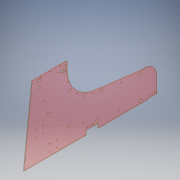
# Autodesk Inventor part: Storage Side Plate
Saved by Autodesk Inventor 2019.4 (Build 234330000, 330)
## iProperties
Created: 2020-01-11
Part Number: Storage Side Plate
Material: Polycarbonate, Smoke
Document SubType Name: Modeling
Designer: admin
Density: 1.2 g/cm^3
Appearance: Polycarbonate - Smoked
Mass: 1698.6 g
Surface Area: 5851.48 cm^2
Volume: 1415.5 cm^3
Author: admin
Autodesk Inventor part; units mm, degrees
ref_plane "YZ Plane" through (0, 0, 0) normal (1, 0, 0) x (0, 1, 0)
ref_plane "XZ Plane" through (0, 0, 0) normal (0, 1, 0) x (-1, 0, 0)
ref_plane "XY Plane" through (0, 0, 0) normal (0, 0, 1) x (1, 0, 0)
sketch "Sketch1" plane through (0, 0, 0) normal (1, 0, 0) x (0, 1, 0)
  arc A0 (273.7291, -166.7427) -> (45.384, -369.2015) centre (273.7291, -396.7427) ccw
  arc A1 (273.7291, 36.4573) -> (-156.3539, -344.8694) centre (273.7291, -396.7427) ccw
  line L0 (45.384, -369.2015) -> (9.2003, -669.2015)
  line L1 (-156.3539, -344.8694) -> (-192.5376, -644.8694)
  line L2 (48.9453, -381.4304) -> (48.9453, -441.4304)
  line L3 (-161.2547, -373.9304) -> (-161.2547, -293.9304)
  arc A2 (9.2003, -669.2015) -> (7.7612, -693.1504) centre (207.7612, -693.1504) ccw
  arc A3 (-192.5376, -644.8694) -> (-195.4388, -693.1504) centre (207.7612, -693.1504) ccw
  line L4 (-195.4388, -693.1504) -> (7.7612, -693.1504)
  line L5 (48.9453, -381.4304) -> (21.7149, -607.1979) construction
  line L6 (-161.2547, -373.9304) -> (-171.9549, -462.646) construction
  line L7 (273.7291, 36.4573) -> (323.7291, 36.4573)
  line L8 (323.7291, 36.4573) -> (323.7291, -166.7427)
  line L9 (323.7291, -166.7427) -> (273.7291, -166.7427)
  dimension "d4" = 203.2
  dimension "d6" = 5
  dimension "d7" = 1.3856
  dimension "d8" = 230
  dimension "d9" = 300
  dimension "d10" = 200
  dimension "d35" = 50
  constraints: 20 end point, 8 point on circle, 5 tangent, 4 centre point, 4 parallel, 2 coincident, 2 horizontal, 2 perpendicular, 1 line through centre
  measures "d4" distance of L7.start L9.end
  measures "d6" distance between parallel lines of L5 L0
  measures "d7" distance between parallel lines of L1 L6
  measures "d8" radius of A0
  measures "d9" vertical distance of L0.start L0.end
  measures "d10" radius of A2
  measures "d35" distance of L7.start L7.end
extrude "Extrusion1" add sketch "Sketch1" along normal blind 5
sketch "Sketch2" plane through (5, 0, 0) normal (1, 0, 0) x (0, 0, -1)
  line L0 (682.6743, -12.5697) -> (412.135, 20.0607) construction
  line L1 (412.135, 20.0607) -> (288.3305, 50.5351) construction
  line L2 (288.3305, 50.5351) -> (190.5511, 132.3607) construction
  line L3 (190.5511, 132.3607) -> (154.7427, 254.7291) construction
  circle A0 centre (682.6743, -12.5697) radius 9.5
  circle A1 centre (412.135, 20.0607) radius 9.5
  circle A2 centre (288.3305, 50.5351) radius 9.5
  circle A3 centre (190.5511, 132.3607) radius 9.5
  circle A4 centre (154.7427, 254.7291) radius 9.5
  line L4 (669.2015, 9.2003) -> (369.2015, 45.384) construction
  circle A5 centre (434.3269, 202.816) radius 88.9 construction
  line L5 (288.3305, 50.5351) -> (296.252, 66.8436) construction
  arc A6 (166.7427, 273.7291) -> (369.2015, 45.384) centre (396.7427, 273.7291) ccw construction
  line L6 (190.5511, 132.3607) -> (207.0464, 143.6702) construction
  line L7 (682.7467, -176.9612) -> (377.4593, -140.1397) construction
  line L8 (377.4593, -140.1397) -> (183.9514, -80.4659) construction
  line L9 (183.9514, -80.4659) -> (41.2141, 63.1735) construction
  line L10 (41.2141, 63.1735) -> (-24.4573, 254.7291) construction
  circle A7 centre (682.7467, -176.9612) radius 9.5
  circle A8 centre (377.4593, -140.1397) radius 9.5
  circle A9 centre (183.9514, -80.4659) radius 9.5
  circle A10 centre (41.2141, 63.1735) radius 9.5
  circle A11 centre (-24.4573, 254.7291) radius 9.5
  line L11 (-24.4573, 254.7291) -> (154.7427, 254.7291) construction
  line L12 (344.8694, -156.3539) -> (644.8694, -192.5376) projected
  line L13 (41.2141, 63.1735) -> (24.0055, 52.9821) construction
  arc A12 (-36.4573, 273.7291) -> (344.8694, -156.3539) centre (396.7427, 273.7291) ccw projected
  line L14 (166.7427, 323.7291) -> (-36.4573, 323.7291) projected
  line L15 (693.1504, -195.4388) -> (693.1504, 7.7612) projected
  line L16 (183.9514, -80.4659) -> (173.6518, -97.6099) construction
  circle A13 centre (155.7427, 296.7291) radius 25.4 construction
  circle A14 centre (-25.4573, 296.7291) radius 25.4 construction
  circle A15 centre (155.7427, 296.7291) radius 9.5
  circle A16 centre (-25.4573, 296.7291) radius 9.5
  circle A17 centre (547.4047, 3.7455) radius 2.75
  circle A18 centre (530.103, -158.5505) radius 2.75
  circle A19 centre (280.7054, -110.3028) radius 2.75
  circle A20 centre (350.2327, 35.2979) radius 2.75
  circle A21 centre (239.4408, 91.4479) radius 2.75
  circle A22 centre (112.5828, -8.6462) radius 2.75
  circle A23 centre (8.3784, 158.9513) radius 2.75
  circle A24 centre (172.6469, 193.5449) radius 2.75
  line L17 (288.3305, 50.5351) -> (183.9514, -80.4659) construction
  point P0 (0, 0)
  dimension "d11" = 272.5
  dimension "d12" = 19
  dimension "d13" = 19
  dimension "d14" = 19
  dimension "d15" = 19
  dimension "d16" = 19
  dimension "d18" = 12
  dimension "d19" = 20
  dimension "d20" = 177.8
  dimension "d22" = 20
  dimension "d23" = 19
  dimension "d24" = 19
  dimension "d25" = 19
  dimension "d26" = 19
  dimension "d28" = 19
  dimension "d29" = 20
  dimension "d34" = 20
  dimension "d36" = 69
  dimension "d37" = 10.4037
  dimension "d38" = 20
  dimension "d39" = 202.5
  dimension "d40" = 127.5
  dimension "d41" = 307.5
  dimension "d42" = 202.5
  dimension "d43" = 202.5
  dimension "d44" = 127.5
  dimension "d46" = 127.5
  dimension "d49" = 12
  dimension "d50" = 50.8
  dimension "d51" = 50.8
  dimension "d52" = 27
  dimension "d53" = 27
  dimension "d54" = 11
  dimension "d55" = 11
  dimension "d56" = 19
  dimension "d57" = 19
  dimension "d58" = 5.5
  dimension "d59" = 5.5
  dimension "d60" = 5.5
  dimension "d61" = 5.5
  dimension "d62" = 5.5
  dimension "d63" = 5.5
  dimension "d64" = 5.5
  dimension "d65" = 5.5
  dimension "d109" = 167.5
  constraints: 28 end point, 23 centre point, 11 coincident, 8 midpoint, 4 line through centre, 4 point on circle, 1 horizontal, 1 parallel
  measures "d11" distance of L0.start L0.end
  measures "d12" diameter of A0
  measures "d13" diameter of A1
  measures "d14" diameter of A2
  measures "d15" diameter of A3
  measures "d16" diameter of A4
  measures "d18" horizontal distance of A6.start L11.end
  measures "d19" distance from line of L4 A1.centre
  measures "d20" diameter of A5
  measures "d22" distance of L6.start L6.end
  measures "d23" diameter of A7
  measures "d24" diameter of A8
  measures "d25" diameter of A9
  measures "d26" diameter of A10
  measures "d28" diameter of A11
  measures "d29" distance between parallel lines of L12 L7
  measures "d34" distance of L13.start L13.end
  measures "d36" distance from line of L14 L11.end
  measures "d37" distance from line of L15 L7.start
  measures "d38" distance of L16.start L16.end
  measures "d39" distance of L7.end L8.end
  measures "d40" distance of L0.end L1.end
  measures "d41" distance of L7.start L7.end
  measures "d42" distance of L8.end L9.end
  measures "d43" distance of L10.end L9.end
  measures "d44" distance of L1.end L2.end
  measures "d46" distance of L2.end L3.end
  measures "d49" horizontal distance of L14.end L10.end
  measures "d50" diameter of A13
  measures "d51" diameter of A14
  measures "d52" distance from line of L14 A13.centre
  measures "d53" distance from line of L14 A14.centre
  measures "d54" horizontal distance of L14.end A14.centre
  measures "d55" horizontal distance of L14.start A13.centre
  measures "d56" diameter of A15
  measures "d57" diameter of A16
  measures "d58" diameter of A17
  measures "d59" diameter of A18
  measures "d60" diameter of A19
  measures "d61" diameter of A20
  measures "d62" diameter of A21
  measures "d63" diameter of A22
  measures "d64" diameter of A23
  measures "d65" diameter of A24
  measures "d109" distance of L5.start L16.start
extrude "Extrusion2" cut sketch "Sketch2" against normal through all
sketch "Sketch3" plane through (5, 0, 0) normal (1, 0, 0) x (0, 0, -1)
  line L0 (166.7427, 323.7291) -> (-36.4573, 323.7291) projected
  line L1 (-36.4573, 323.7291) -> (-76.4573, 323.7291)
  line L2 (-76.4573, 323.7291) -> (-76.4573, -195.4388)
  arc A0 (644.8694, -192.5376) -> (693.1504, -195.4388) centre (693.1504, 207.7612) ccw projected
  line L3 (-76.4573, -195.4388) -> (693.1504, -195.4388)
  arc A1 (-36.4573, 273.7291) -> (344.8694, -156.3539) centre (396.7427, 273.7291) ccw projected
  line L4 (344.8694, -156.3539) -> (644.8694, -192.5376) projected
  line L5 (-36.4573, 323.7291) -> (-36.4573, 273.7291) projected
  point P0 (0, 0)
  dimension "d66" = 40
  constraints: 6 end point, 2 perpendicular, 1 horizontal, 1 tangent
  measures "d66" distance of L0.end L1.end
extrude "Extrusion3" add sketch "Sketch3" against normal up to surface (5 mm away)
sketch "Sketch4" plane through (5, 0, 0) normal (1, 0, 0) x (0, 0, -1)
  line L0 (299.6427, -195.4388) -> (385.6427, -195.4388)
  line L1 (385.6427, -195.4388) -> (385.6427, -163.2388)
  line L2 (385.6427, -163.2388) -> (299.6427, -163.2388)
  line L3 (299.6427, -163.2388) -> (299.6427, -195.4388)
  line L4 (-76.4573, 323.7291) -> (-76.4573, -195.4388) projected
  line L5 (-76.4573, -195.4388) -> (693.1504, -195.4388) projected
  point P0 (0, 0)
  dimension "d69" = 376.1
  dimension "d70" = 32.2
  dimension "d71" = 86
  constraints: 8 end point, 2 parallel, 1 collinear, 1 horizontal, 1 perpendicular
  measures "d69" distance between parallel lines of L3 L4
  measures "d70" distance of L2.end L0.start
  measures "d71" distance of L1.end L2.end
extrude "Extrusion4" cut sketch "Sketch4" against normal through all
fillet "Fillet1" radius 3 2 edges at (2.5, -163.2388, -299.6427) (2.5, -163.2388, -385.6427)
thicken "Thicken1" operation add thickness 2.2 both sides no extend neighbours yes toward (0, 1, 0) faces at (3.3333, -195.4388, -48.9094)
thicken "Thicken2" operation add thickness 2.2 both sides no extend neighbours yes toward (0, 1, 0) faces at (1.6667, -195.4388, -488.1453)
sketch "Sketch5" plane through (5, 0, 0) normal (1, 0, 0) x (0, 0, -1)
  line L0 (693.1504, 7.7612) -> (793.1504, 7.7612)
  line L1 (793.1504, 7.7612) -> (793.1504, -188.2388)
  line L2 (793.1504, -188.2388) -> (732.1504, -188.2388)
  line L3 (732.1504, -188.2388) -> (732.1504, -193.2388)
  line L4 (385.6427, -193.2388) -> (693.1504, -193.2388) projected
  line L5 (732.1504, -193.2388) -> (693.1504, -193.2388)
  line L6 (693.1504, -193.2388) -> (693.1504, 7.7612)
  point P0 (0, 0)
  dimension "d79" = 5
  dimension "d80" = 100
  dimension "d81" = 39
  constraints: 12 end point, 4 perpendicular, 1 horizontal, 1 vertical
  measures "d79" distance of L2.end L3.end
  measures "d80" distance of L0.start L0.end
  measures "d81" distance of L3.end L4.end
extrude "Extrusion5" add sketch "Sketch5" against normal up to surface (5 mm away)
fillet "Fillet2" radius 3 1 edges at (2.5, -188.2388, -732.1504)
fillet "Fillet3" radius 80 1 edges at (2.5, 7.7612, -793.1504)
sketch "Sketch6" plane through (0, 0, 0) normal (-1, 0, 0) x (0, 0, 1)
  circle A0 centre (-352.6427, -150.2388) radius 2.75 projected
  circle A1 centre (-332.6427, -150.2388) radius 2.75 projected
  circle A2 centre (-312.6427, -150.2388) radius 2.75 projected
  point P0 (0, 0)
extrude "Extrusion6" cut sketch "Sketch6" against normal through all
sketch "Sketch7" plane through (5, 0, 0) normal (1, 0, 0) x (0, 0, -1)
  circle A0 centre (743.1504, -175.2388) radius 2.75 projected
  circle A1 centre (763.1504, -175.2388) radius 2.75 projected
  circle A2 centre (783.1504, -175.2388) radius 2.75 projected
  point P0 (0, 0)
extrude "Extrusion7" cut sketch "Sketch7" against normal through all
sketch "Sketch8" plane through (5, 0, 0) normal (1, 0, 0) x (0, 0, -1)
  line L0 (166.7427, 323.7291) -> (-76.4573, 323.7291) projected
  line L1 (-76.4573, 323.7291) -> (-134.8573, -193.2388)
  line L2 (299.6427, -193.2388) -> (-76.4573, -193.2388) projected
  line L3 (-134.8573, -193.2388) -> (-76.4573, -193.2388)
  line L4 (-76.4573, -193.2388) -> (-76.4573, 323.7291)
  line L5 (-76.4573, -193.2388) -> (299.6427, -193.2388) projected
  point P0 (0, 0)
  dimension "d90" = 58.4
  constraints: 6 end point, 1 collinear, 1 perpendicular
  measures "d90" distance of L2.end L1.end
extrude "Extrusion8" add sketch "Sketch8" against normal up to surface (5 mm away)
sketch "Sketch9" plane through (5, 0, 0) normal (1, 0, 0) x (0, 0, -1)
  circle A0 centre (-16.4573, 313.7291) radius 2.75 projected
  circle A1 centre (53.5427, 313.7291) radius 2.75 projected
  circle A2 centre (123.5427, 313.7291) radius 2.75 projected
  circle A3 centre (312.6427, -150.2388) radius 2.75 projected
  circle A4 centre (332.6427, -150.2388) radius 2.75 projected
  circle A5 centre (352.6427, -150.2388) radius 2.75 projected
  circle A6 centre (743.1504, -175.2388) radius 2.75 projected
  circle A7 centre (763.1504, -175.2388) radius 2.75 projected
  circle A8 centre (783.1504, -175.2388) radius 2.75 projected
  point P0 (0, 0)
extrude "Extrusion9" cut sketch "Sketch9" against normal through all contours A0 | A1 | A2
sketch "Sketch10" plane through (5, 0, 0) normal (1, 0, 0) x (0, 0, -1)
  circle A0 centre (73.275, -143.7666) radius 9.5 construction
  circle A1 centre (183.9514, -80.4659) radius 9.5 projected
  line L0 (73.275, -143.7666) -> (183.9514, -80.4659) construction
  line L1 (-134.8573, -193.2388) -> (299.6427, -193.2388) projected
  line L2 (48.275, -168.7666) -> (98.275, -168.7666) construction
  line L3 (98.275, -168.7666) -> (98.275, -118.7666) construction
  line L4 (98.275, -118.7666) -> (48.275, -118.7666) construction
  line L5 (48.275, -118.7666) -> (48.275, -168.7666) construction
  line L6 (48.275, -168.7666) -> (98.275, -118.7666) construction
  line L7 (98.275, -168.7666) -> (48.275, -118.7666) construction
  circle A2 centre (48.275, -118.7666) radius 2.2
  circle A3 centre (98.275, -118.7666) radius 2.2
  circle A4 centre (48.275, -168.7666) radius 2.2
  circle A5 centre (98.275, -168.7666) radius 2.2
  circle A6 centre (190.5511, 132.3607) radius 9.5 projected
  line L8 (73.275, -143.7666) -> (190.5511, 132.3607) construction
  circle A7 centre (-25.4573, -10.7709) radius 9.5 construction
  line L9 (-50.4573, -35.7709) -> (-0.4573, -35.7709) construction
  line L10 (-0.4573, -35.7709) -> (-0.4573, 14.2291) construction
  line L11 (-0.4573, 14.2291) -> (-50.4573, 14.2291) construction
  line L12 (-50.4573, 14.2291) -> (-50.4573, -35.7709) construction
  line L13 (-50.4573, -35.7709) -> (-0.4573, 14.2291) construction
  line L14 (-0.4573, -35.7709) -> (-50.4573, 14.2291) construction
  circle A8 centre (-50.4573, 14.2291) radius 2.2
  circle A9 centre (-0.4573, 14.2291) radius 2.2
  circle A10 centre (-50.4573, -35.7709) radius 2.2
  circle A11 centre (-0.4573, -35.7709) radius 2.2
  circle A12 centre (-25.4573, 296.7291) radius 9.5 projected
  line L15 (-25.4573, -10.7709) -> (-25.4573, 296.7291) construction
  point P0 (0, 0)
  dimension "d98" = 19
  dimension "d99" = 127.5
  dimension "d101" = 4.4
  dimension "d102" = 4.4
  dimension "d103" = 4.4
  dimension "d104" = 4.4
  dimension "d105" = 50
  dimension "d108" = 300
  dimension "d110" = 19
  dimension "d111" = 4.4
  dimension "d112" = 4.4
  dimension "d113" = 4.4
  dimension "d114" = 4.4
  dimension "d115" = 50
  dimension "d116" = 307.5
  constraints: 30 end point, 10 centre point, 8 coincident, 4 midpoint, 4 parallel, 4 perpendicular, 2 horizontal, 1 vertical
  measures "d98" diameter of A0
  measures "d99" distance of L0.start L0.end
  measures "d101" diameter of A2
  measures "d102" diameter of A3
  measures "d103" diameter of A4
  measures "d104" diameter of A5
  measures "d105" distance of L2.end L3.end
  measures "d108" distance of L0.start L8.end
  measures "d110" diameter of A7
  measures "d111" diameter of A8
  measures "d112" diameter of A9
  measures "d113" diameter of A10
  measures "d114" diameter of A11
  measures "d115" distance of L10.start L10.end
  measures "d116" distance of L15.start L15.end
extrude "Extrusion10" cut sketch "Sketch10" against normal through all contours A2 | A3 | A4 | A5 | A8 | A9 | A10 | A11
sketch "Sketch11" plane through (5, 0, 0) normal (1, 0, 0) x (0, 0, -1)
  circle A0 centre (-25.4573, 296.7291) radius 9.5 projected
  line L0 (-25.4573, 296.7291) -> (130.9409, 278.1315) construction
  circle A1 centre (130.9409, 278.1315) radius 9.5
  circle A2 centre (155.7427, 296.7291) radius 9.5 projected
  line L1 (130.9409, 278.1315) -> (155.7427, 296.7291) construction
  circle A3 centre (108.5983, 280.7883) radius 2.2
  circle A4 centre (153.2835, 275.4748) radius 2.2
  line L2 (153.2835, 275.4748) -> (130.9409, 278.1315) construction
  point P0 (0, 0)
  dimension "d117" = 19
  dimension "d118" = 157.5
  dimension "d119" = 31
  dimension "d122" = 4.4
  dimension "d123" = 4.4
  dimension "d124" = 22.5
  dimension "d125" = 22.5
  constraints: 6 end point, 3 centre point, 1 coincident, 1 collinear, 1 point on line
  measures "d117" diameter of A1
  measures "d118" distance of L0.start L0.end
  measures "d119" distance of L1.start L1.end
  measures "d122" diameter of A3
  measures "d123" diameter of A4
  measures "d124" distance of L0.end A3.centre
  measures "d125" distance of L0.end L2.start
extrude "Extrusion11" cut sketch "Sketch11" against normal through all contours A1 | A3 | A4
body "Solid1"
